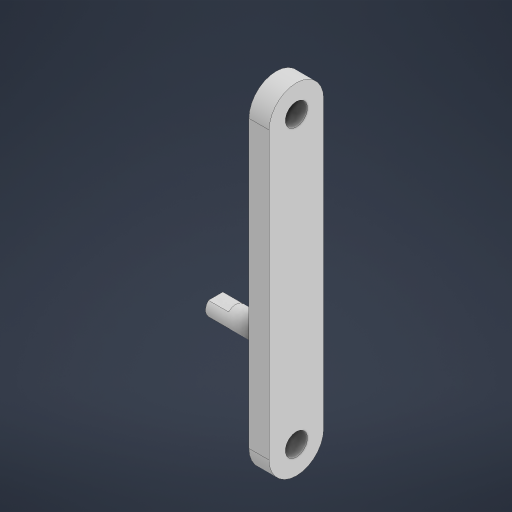
# Autodesk Inventor part: gunholder
Saved by Autodesk Inventor 2024 (Build 280153000, 153)
## iProperties
Created: 2023-06-15
Part Number: gunholder
Material: 일반
Document SubType Name: Modeling
Designer: 6gioc
Density: 1 g/cm^3
Appearance: 기본값
Author: 6gioc
## iProperties of the stored document gunholder_3D 인쇄.ipt
Created: 2023-06-20
Part Number: gunholder_3D 인쇄
Material: 일반
Document SubType Name: Modeling
Designer: 6gioc
Density: 1 g/cm^3
Appearance: 기본값
Author: 6gioc
Autodesk Inventor part; units mm, degrees
ref_plane "YZ Plane" through (0, 0, 0) normal (1, 0, 0) x (0, 1, 0)
ref_plane "XZ Plane" through (0, 0, 0) normal (0, 1, 0) x (-1, 0, 0)
ref_plane "XY Plane" through (0, 0, 0) normal (0, 0, 1) x (1, 0, 0)
sketch "스케치4" plane through (0, 0, 0) normal (1, 0, 0) x (0, 1, 0)
  circle A0 centre (0, 0) radius 2.75
  circle A1 centre (0, 0) radius 6.75
  line L0 (0, 0) -> (-70.8, 0) construction
  line L1 (0, 0) -> (70.8, 0) construction
  circle A2 centre (-70.8, 0) radius 2.75
  circle A3 centre (-70.8, 0) radius 6.75
  line L2 (0, 6.75) -> (-70.8, 6.75)
  line L3 (-70.8, -6.75) -> (0, -6.75)
  circle A4 centre (-50.7564, 0) radius 2.5
  circle A5 centre (-50.7564, 0) radius 1.75
  line L4 (-49.0064, 0) -> (-49.0064, 1.7854)
  line L5 (-49.0064, 0) -> (-49.0064, -1.7854)
  line L6 (-52.5064, 0) -> (-52.5064, -1.7854)
  line L7 (-52.5064, 0) -> (-52.5064, 1.7854)
  dimension "d29" = 5.5
  dimension "d30" = 13.5
  dimension "d31" = 70.8
  dimension "d32" = 180
  dimension "d33" = 5.5
  dimension "d34" = 13.5
  dimension "d35" = 5
  dimension "d36" = 3.5
  constraints: 16 end point, 10 point on circle, 6 centre point, 5 coincident, 4 point on line, 4 tangent, 3 horizontal, 1 collinear, 1 parallel, 1 vertical
  measures "d29" diameter of A0
  measures "d30" diameter of A1
  measures "d31" distance of L0.start L0.end
  measures "d32" angle of L0 L1
  measures "d33" diameter of A2
  measures "d34" diameter of A3
  measures "d35" diameter of A4
  measures "d36" diameter of A5
extrude "돌출6" add sketch "스케치4" along normal blind 5 contours A1 | A1 L3 A3 L2 | A3 | A4 L5 L4 | L4 A5 L7 A4 | A4 L6 A5 L5 | L7 L6 A4 | A5
extrude "돌출7" add sketch "스케치4" against normal blind 15 contours L4 A5 L7 A4 | A4 L6 A5 L5 | A5
extrude "돌출8" add sketch "스케치4" against normal blind 10 contours A4 L5 L4 | L7 L6 A4
